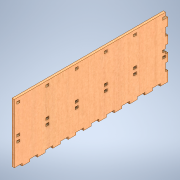
# Autodesk Inventor part: DoosjeRechterkant
Saved by Autodesk Inventor 2021 (Build 250183000, 183)
## iProperties
Created: 2021-03-11
Part Number: DoosjeRechterkant
Material: Wood (Cherry)
Document SubType Name: Modeling
Designer: ZiweZhang
Density: 0.63 g/cm^3
Appearance: Cherry - Natural Low Gloss
Author: ZiweZhang
Autodesk Inventor part; units mm, degrees
ref_plane "YZ Plane" through (0, 0, 0) normal (1, 0, 0) x (0, 1, 0)
ref_plane "XZ Plane" through (0, 0, 0) normal (0, 1, 0) x (-1, 0, 0)
ref_plane "XY Plane" through (0, 0, 0) normal (0, 0, 1) x (1, 0, 0)
sketch "Sketch1" plane through (0, 0, 0) normal (1, 0, 0) x (0, 1, 0)
  line L0 (0, 0) -> (77, 0)
  line L1 (77, 0) -> (77, -200)
  line L2 (77, -200) -> (0, -200)
  line L3 (0, -200) -> (0, 0)
  dimension "d0" = 77
  dimension "d1" = 200
  constraints: 8 end point, 2 parallel, 1 horizontal, 1 perpendicular
  measures "d0" distance of L1.end L2.end
  measures "d1" distance of L0.end L1.end
extrude "Extrusion1" add sketch "Sketch1" along normal blind 3
sketch "Sketch2" plane through (3, 0, 0) normal (1, 0, 0) x (0, 0, -1)
  line L0 (0, 0) -> (10, 0)
  line L1 (0, 0) -> (200, 0) projected
  line L2 (10, 0) -> (10, -3)
  line L3 (10, -3) -> (20, -3)
  line L4 (20, -3) -> (20, 0)
  line L5 (0, 0) -> (200, 0) projected
  line L6 (30, -3) -> (40, -3)
  line L7 (20, 0) -> (30, 0)
  line L8 (30, 0) -> (30, -3)
  line L9 (40, -3) -> (40, 0)
  line L10 (50, -3) -> (60, -3)
  line L11 (40, 0) -> (50, 0)
  line L12 (50, 0) -> (50, -3)
  line L13 (60, -3) -> (60, 0)
  line L14 (70, -3) -> (80, -3)
  line L15 (60, 0) -> (70, 0)
  line L16 (70, 0) -> (70, -3)
  line L17 (80, -3) -> (80, 0)
  line L18 (90, -3) -> (100, -3)
  line L19 (80, 0) -> (90, 0)
  line L20 (90, 0) -> (90, -3)
  line L21 (100, -3) -> (100, 0)
  line L22 (110, -3) -> (120, -3)
  line L23 (100, 0) -> (110, 0)
  line L24 (110, 0) -> (110, -3)
  line L25 (120, -3) -> (120, 0)
  line L26 (130, -3) -> (140, -3)
  line L27 (120, 0) -> (130, 0)
  line L28 (130, 0) -> (130, -3)
  line L29 (140, -3) -> (140, 0)
  line L30 (150, -3) -> (160, -3)
  line L31 (140, 0) -> (150, 0)
  line L32 (150, 0) -> (150, -3)
  line L33 (160, -3) -> (160, 0)
  line L34 (170, -3) -> (180, -3)
  line L35 (160, 0) -> (170, 0)
  line L36 (170, 0) -> (170, -3)
  line L37 (180, -3) -> (180, 0)
  line L38 (190, -3) -> (200, -3)
  line L39 (180, 0) -> (190, 0)
  line L40 (190, 0) -> (190, -3)
  line L41 (200, -3) -> (200, 0)
  line L42 (0, 0) -> (0, 10)
  line L43 (200, 77) -> (0, 77) projected
  line L44 (200, 0) -> (200, 77) projected
  line L45 (200, 0) -> (200, 10)
  line L46 (197, 10) -> (197, 20)
  line L47 (197, 20) -> (200, 20)
  line L48 (200, 30) -> (197, 30)
  line L49 (197, 30) -> (197, 40)
  line L50 (197, 40) -> (200, 40)
  line L51 (200, 40) -> (200, 50)
  line L52 (200, 50) -> (197, 50)
  line L53 (197, 50) -> (197, 60)
  line L54 (197, 60) -> (200, 60)
  line L55 (200, 60) -> (200, 70)
  line L56 (200, 70) -> (197, 70)
  line L57 (197, 70) -> (197, 77)
  line L58 (200, 10) -> (197, 10)
  line L59 (200, 20) -> (200, 30)
  line L60 (3, 77) -> (197, 77)
  line L61 (0, 77) -> (0, 0) projected
  line L62 (0, 0) -> (0, 77)
  line L63 (0, 77) -> (3, 77)
  point P0 (0, 70)
  dimension "d9" = 20
  dimension "d25" = 10
  constraints: 118 end point, 17 point on line, 8 perpendicular, 3 collinear, 2 horizontal, 2 vertical, 1 parallel, 81 other
  measures "d9" distance of L2.end L6.start
  measures "d25" distance of L46.start L46.end
extrude "Extrusion2" cut sketch "Sketch2" against normal blind 3 contours L42 L61 L43 L57 L56 L44 L54 L53 L52 L50 L49 L48 L47 L46 L58 L1 L0 keep common part
sketch "Sketch3" plane through (3, 0, 0) normal (1, 0, 0) x (0, 0, -1)
  line L0 (0, 0) -> (10, 0)
  line L1 (0, 0) -> (200, 0)
  line L2 (10, 0) -> (10, -3)
  line L3 (10, -3) -> (20, -3)
  line L4 (20, -3) -> (20, 0)
  line L5 (30, -3) -> (40, -3)
  line L6 (20, 0) -> (30, 0)
  line L7 (30, 0) -> (30, -3)
  line L8 (40, -3) -> (40, 0)
  line L9 (50, -3) -> (60, -3)
  line L10 (40, 0) -> (50, 0)
  line L11 (50, 0) -> (50, -3)
  line L12 (60, -3) -> (60, 0)
  line L13 (70, -3) -> (80, -3)
  line L14 (60, 0) -> (70, 0)
  line L15 (70, 0) -> (70, -3)
  line L16 (80, -3) -> (80, 0)
  line L17 (90, -3) -> (100, -3)
  line L18 (80, 0) -> (90, 0)
  line L19 (90, 0) -> (90, -3)
  line L20 (100, -3) -> (100, 0)
  line L21 (110, -3) -> (120, -3)
  line L22 (100, 0) -> (110, 0)
  line L23 (110, 0) -> (110, -3)
  line L24 (120, -3) -> (120, 0)
  line L25 (130, -3) -> (140, -3)
  line L26 (120, 0) -> (130, 0)
  line L27 (130, 0) -> (130, -3)
  line L28 (140, -3) -> (140, 0)
  line L29 (150, -3) -> (160, -3)
  line L30 (140, 0) -> (150, 0)
  line L31 (150, 0) -> (150, -3)
  line L32 (160, -3) -> (160, 0)
  line L33 (170, -3) -> (180, -3)
  line L34 (160, 0) -> (170, 0)
  line L35 (170, 0) -> (170, -3)
  line L36 (180, -3) -> (180, 0)
  line L37 (190, -3) -> (200, -3)
  line L38 (180, 0) -> (190, 0)
  line L39 (190, 0) -> (190, -3)
  line L40 (10, 0) -> (10, -3)
  line L41 (20, -3) -> (20, 0)
  line L42 (0, 0) -> (30, 0)
  line L43 (40, 0) -> (200, 0)
  line L44 (0, 0) -> (200, 0) projected
  line L45 (200, -3) -> (200, 0)
  dimension "d28" = 10
  dimension "d29" = 3
  dimension "d30" = 10
  dimension "d31" = 20
  constraints: 88 end point, 3 perpendicular, 1 collinear, 1 point on line, 1 vertical, 5 other
  measures "d28" distance of L0.start L0.end
  measures "d29" distance of L0.end L2.end
  measures "d30" distance of L2.end L4.start
  measures "d31" distance of L2.end L7.end
extrude "Extrusion3" add sketch "Sketch3" against normal blind 3
sketch "Sketch4" plane through (3, 0, 0) normal (1, 0, 0) x (0, 0, -1)
  line L0 (197, 70) -> (197, 77) projected
  line L1 (197, 73) -> (193, 73)
  line L2 (193, 73) -> (193, 70)
  line L3 (193, 70) -> (197, 70)
  line L4 (197, 70) -> (197, 73)
  line L5 (159, 73) -> (155, 73)
  line L6 (155, 73) -> (155, 70)
  line L7 (155, 70) -> (159, 70)
  line L8 (159, 70) -> (159, 73)
  line L9 (197, 36) -> (193, 36)
  line L10 (193, 36) -> (193, 33)
  line L11 (193, 33) -> (197, 33)
  line L12 (197, 33) -> (197, 36)
  line L13 (159, 36) -> (155, 36)
  line L14 (155, 36) -> (155, 33)
  line L15 (155, 33) -> (159, 33)
  line L16 (159, 33) -> (159, 36)
  line L17 (121, 73) -> (117, 73)
  line L18 (117, 73) -> (117, 70)
  line L19 (117, 70) -> (121, 70)
  line L20 (121, 70) -> (121, 73)
  line L21 (121, 36) -> (117, 36)
  line L22 (117, 36) -> (117, 33)
  line L23 (117, 33) -> (121, 33)
  line L24 (121, 33) -> (121, 36)
  line L25 (83, 73) -> (79, 73)
  line L26 (79, 73) -> (79, 70)
  line L27 (79, 70) -> (83, 70)
  line L28 (83, 70) -> (83, 73)
  line L29 (83, 36) -> (79, 36)
  line L30 (79, 36) -> (79, 33)
  line L31 (79, 33) -> (83, 33)
  line L32 (83, 33) -> (83, 36)
  line L33 (45, 73) -> (41, 73)
  line L34 (41, 73) -> (41, 70)
  line L35 (41, 70) -> (45, 70)
  line L36 (45, 70) -> (45, 73)
  line L37 (45, 36) -> (41, 36)
  line L38 (41, 36) -> (41, 33)
  line L39 (41, 33) -> (45, 33)
  line L40 (45, 33) -> (45, 36)
  line L41 (159, 33) -> (159, 36)
  line L42 (155, 33) -> (159, 33)
  line L43 (159, 36) -> (155, 36)
  line L44 (155, 36) -> (155, 33)
  line L45 (121, 33) -> (121, 36)
  line L46 (117, 33) -> (121, 33)
  line L47 (121, 36) -> (117, 36)
  line L48 (117, 36) -> (117, 33)
  line L49 (83, 33) -> (83, 36)
  line L50 (79, 33) -> (83, 33)
  line L51 (83, 36) -> (79, 36)
  line L52 (79, 36) -> (79, 33)
  line L53 (45, 33) -> (45, 36)
  line L54 (41, 33) -> (45, 33)
  line L55 (45, 36) -> (41, 36)
  line L56 (41, 36) -> (41, 33)
  line L57 (197, 26) -> (197, 29)
  line L58 (193, 26) -> (197, 26)
  line L59 (197, 29) -> (193, 29)
  line L60 (193, 29) -> (193, 26)
  line L61 (159, 26) -> (159, 29)
  line L62 (155, 26) -> (159, 26)
  line L63 (159, 29) -> (155, 29)
  line L64 (155, 29) -> (155, 26)
  line L65 (121, 26) -> (121, 29)
  line L66 (117, 26) -> (121, 26)
  line L67 (121, 29) -> (117, 29)
  line L68 (117, 29) -> (117, 26)
  line L69 (83, 26) -> (83, 29)
  line L70 (79, 26) -> (83, 26)
  line L71 (83, 29) -> (79, 29)
  line L72 (79, 29) -> (79, 26)
  line L73 (45, 26) -> (45, 29)
  line L74 (41, 26) -> (45, 26)
  line L75 (45, 29) -> (41, 29)
  line L76 (41, 29) -> (41, 26)
  line L77 (7, 73) -> (3, 73)
  line L78 (3, 73) -> (3, 70)
  line L79 (3, 70) -> (7, 70)
  line L80 (7, 70) -> (7, 73)
  line L81 (7, 36) -> (3, 36)
  line L82 (3, 36) -> (3, 33)
  line L83 (3, 33) -> (7, 33)
  line L84 (7, 33) -> (7, 36)
  line L85 (7, 33) -> (7, 36)
  line L86 (3, 33) -> (7, 33)
  line L87 (7, 36) -> (3, 36)
  line L88 (3, 36) -> (3, 33)
  line L89 (7, 26) -> (7, 29)
  line L90 (3, 26) -> (7, 26)
  line L91 (7, 29) -> (3, 29)
  line L92 (3, 29) -> (3, 26)
  line L93 (197, 77) -> (0, 77) projected
  point P0 (0, 0)
  dimension "d34" = 4
  dimension "d35" = 3
  dimension "d38" = 38
  dimension "d41" = 37
  dimension "d48" = 38
  dimension "d51" = 7
  dimension "d54" = 4
  constraints: 184 end point, 4 collinear, 3 horizontal, 2 parallel, 2 vertical, 1 perpendicular, 1 point on line, 172 other
  measures "d34" distance of L3.end L2.end
  measures "d35" distance of L2.end L1.end
  measures "d38" distance of L1.start L5.start
  measures "d41" distance of L1.start L9.start
  measures "d48" distance of L11.end L41.start
  measures "d51" distance of L11.end L57.start
  measures "d54" distance between parallel lines of L93 L1
extrude "Extrusion4" cut sketch "Sketch4" against normal through all
body "Solid1"
